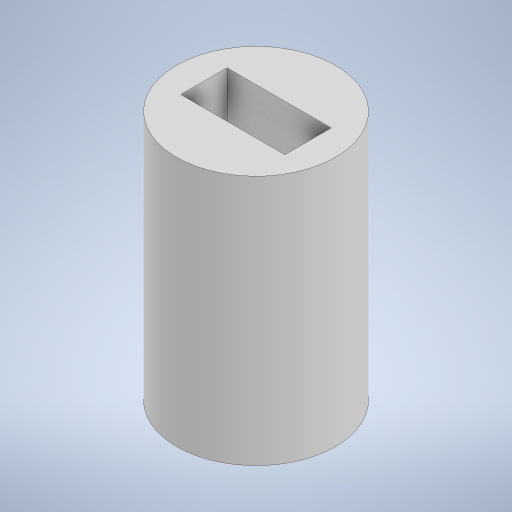
# Autodesk Inventor part: encoder_magnet_holder2
Saved by Autodesk Inventor 2023 (Build 270158000, 158)
## iProperties
Created: 2023-02-14
Part Number: encoder_magnet_holder2
Material: Generic
Document SubType Name: Modeling
Designer: jxl19
Density: 1 g/cm^3
Appearance: Default
Author: jxl19
## iProperties of the stored document encoder_magnet_holder_3DPrint.ipt
Created: 2023-02-14
Part Number: encoder_magnet_holder_3DPrint
Material: Generic
Document SubType Name: Modeling
Designer: jxl19
Density: 1 g/cm^3
Appearance: Default
Author: jxl19
Autodesk Inventor part; units mm, degrees
ref_plane "YZ Plane" through (0, 0, 0) normal (1, 0, 0) x (0, 1, 0)
ref_plane "XZ Plane" through (0, 0, 0) normal (0, 1, 0) x (-1, 0, 0)
ref_plane "XY Plane" through (0, 0, 0) normal (0, 0, 1) x (1, 0, 0)
sketch "Sketch1" plane through (0, 0, 0) normal (0, 1, 0) x (-1, 0, 0)
  circle A0 centre (0, 0) radius 4.125
  dimension "d0" = 8.25
  constraints: 1 centre point, 1 coincident
  measures "d0" diameter of A0
extrude "Extrusion1" add sketch "Sketch1" along normal blind 13
sketch "Sketch2" plane through (0, 0, 0) normal (0, -1, 0) x (1, 0, 0)
  circle A0 centre (0, 0) radius 1
  dimension "d3" = 2
  constraints: 1 centre point, 1 coincident
  measures "d3" diameter of A0
extrude "Extrusion2" cut sketch "Sketch2" against normal blind 8
sketch "Sketch3" plane through (0, 13, 0) normal (0, 1, 0) x (1, 0, 0)
  line L0 (-2.7, -1.2) -> (2.7, -1.2)
  line L1 (2.7, -1.2) -> (2.7, 1.2)
  line L2 (2.7, 1.2) -> (-2.7, 1.2)
  line L3 (-2.7, 1.2) -> (-2.7, -1.2)
  line L4 (-2.7, -1.2) -> (2.7, 1.2) construction
  line L5 (2.7, -1.2) -> (-2.7, 1.2) construction
  point P0 (0, 0)
  dimension "d6" = 2.4
  dimension "d7" = 5.4
  constraints: 12 end point, 2 midpoint, 2 parallel, 1 horizontal, 1 perpendicular
  measures "d6" distance of L2.end L0.start
  measures "d7" distance of L1.end L2.end
extrude "Extrusion3" cut sketch "Sketch3" against normal blind 5
body "Solid1"
